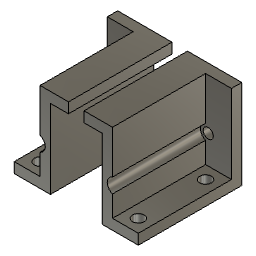
USB_Hub_Mount (Autodesk Fusion 360 design; units mm, degrees)
Autodesk Fusion 360 part; units mm, degrees
note: some values were not read from the file. Set by a fixed rule: which sketch regions a step uses.
sketch "Sketch1" plane through (0, 0, 0) normal (0, 1, 0) x (1, 0, 0)
  line L0 (0, 0) -> (0, -30.5)
  line L1 (0, -30.5) -> (-7, -30.5)
  line L2 (-7, -30.5) -> (-7, -34.5)
  line L3 (-7, -34.5) -> (4, -34.5)
  line L4 (4, -34.5) -> (4, -4)
  line L5 (4, -4) -> (14, -4)
  line L6 (14, -4) -> (14, 0)
  line L7 (14, 0) -> (0, 0)
  line L8 (5, 0) -> (5, -15) construction
  circle A0 centre (5, -15) radius 1.95
  line L9 (4, -34.5) -> (14, -34.5)
  line L10 (14, -34.5) -> (14, -4)
  line L11 (14, -4) -> (4, -4) construction
  line L12 (4, -4) -> (4, -34.5) construction
  circle A1 centre (5, -15) radius 3
  dimension "d1" = 30.5
  dimension "d2" = 4
  dimension "d3" = 7
  dimension "d4" = 4
  dimension "d5" = 4
  dimension "d6" = 10
  dimension "d7" = 3.9
  dimension "d8" = 15
  dimension "d9" = 5
  dimension "d10" = 6
  constraint coincident L0.start L7.end
  constraint vertical L0
  constraint perpendicular L0 L1
  constraint perpendicular L1 L2
  constraint perpendicular L2 L3
  constraint perpendicular L3 L4
  constraint perpendicular L4 L5
  constraint perpendicular L5 L6
  constraint horizontal L7
  constraint coincident L7 L8.start
  constraint perpendicular L7 L8
  constraint coincident L8.end A0.centre
  constraint horizontal L9
  constraint vertical L10
  constraint horizontal L11
  constraint vertical L12
  constraint concentric A0 A1
  measures "d1" distance of L0.start L0.end
  measures "d2" distance of L1.end L2.end
  measures "d3" distance of L0.end L1.end
  measures "d4" horizontal distance of L0.start L4.end
  measures "d5" distance of L5.end L6.end
  measures "d6" distance of L4.end L5.end
  measures "d7" diameter of A0
  measures "d8" distance of L8.start L8.end
  measures "d9" distance of L0 L8.end
  measures "d10" diameter of A1
extrude "Extrude1" add sketch "Sketch1" against normal blind 4 contours L0 L1 L2 L3 L4 L5 L6 L7 A1 | L4 L5 L9 L10 A1 | L4 A0 A1 | L4 A0 A1 makes body 1
extrude "Extrude2" add sketch "Sketch1" against normal blind 40 contours L0 L1 L2 L3 L4 L5 L6 L7 A1 bodies 1
sketch "Sketch2" plane through (0, 0, 4) normal (0, 0, 1) x (-1, 0, 0)
  line L0 (-14, 4) -> (-4, 4)
  line L1 (-4, 4) -> (-4, 40)
  line L2 (-4, 40) -> (-14, 40)
  line L3 (-14, 40) -> (-14, 4)
  line L4 (-9, 4) -> (-9, 40) construction
  circle A0 centre (-9, 9) radius 5 construction
  circle A1 centre (-9, 35) radius 5 construction
  circle A2 centre (-9, 9) radius 2.25
  circle A3 centre (-9, 35) radius 2.25
  dimension "d15" = 10
  dimension "d17" = 5
  dimension "d18" = 5
  dimension "d19" = 4.5
  constraint midpoint L0 L4.start
  constraint midpoint L2 L4.end
  constraint coincident L4 A0.centre
  constraint coincident L4 A1.centre
  constraint concentric A0 A2
  constraint concentric A1 A3
  constraint equal A2 A3
  constraint equal A0 A1
  measures "d15" diameter of A0
  measures "d17" distance of L4.end A1.centre
  measures "d18" distance of L4.start A0.centre
  measures "d19" diameter of A2
extrude "Extrude3" cut sketch "Sketch2" against normal blind 8 contours A2 | A3 bodies 1
mirror "Mirror1" about plane through (0, 0, 0) normal (1, 0, 0) of bodies 1 makes body 2
move_body "Move1" bodies 2 to x (1, 0, 0) y (0, 1, 0) z (0, 0, 1) at (-20, 0, 0)
named bodies: "USB_Hub_Mount_right", "USB_Hub_Mount_left"
